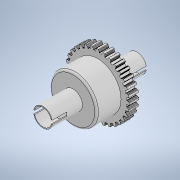
# Autodesk Inventor part: Дифференциал
Saved by Autodesk Inventor 2020 (Build 240168000, 168)
## iProperties
Created: 2021-05-23
Part Number: Дифференциал
Material: Типовые
Document SubType Name: Modeling
Designer: Антон
Density: 1 g/cm^3
Appearance: По умолчанию
Author: Антон
Autodesk Inventor part; units mm, degrees
ref_plane "YZ Plane" through (0, 0, 0) normal (1, 0, 0) x (0, 1, 0)
ref_plane "XZ Plane" through (0, 0, 0) normal (0, 1, 0) x (-1, 0, 0)
sketch "Эскиз1" plane through (0, 0, 0) normal (0, 0, 1) x (1, 0, 0)
  line L0 (32.4043, 17.9453) -> (32.4686, 17.9378)
  line L1 (32.4686, 17.9378) -> (32.5329, 17.9288)
  line L2 (32.5329, 17.9288) -> (32.6618, 17.9069)
  line L3 (32.6618, 17.9069) -> (32.9201, 17.8497)
  line L4 (32.9201, 17.8497) -> (33.1788, 17.7769)
  line L5 (33.1788, 17.7769) -> (33.4377, 17.69)
  line L6 (33.4377, 17.69) -> (33.6965, 17.5903)
  line L7 (33.6965, 17.5903) -> (33.9549, 17.4785)
  line L8 (33.9549, 17.4785) -> (33.9549, 16.4837)
  line L9 (33.9549, 16.4837) -> (33.6965, 16.3719)
  line L10 (33.6965, 16.3719) -> (33.4377, 16.2722)
  line L11 (33.4377, 16.2722) -> (33.1788, 16.1854)
  line L12 (33.1788, 16.1854) -> (32.9201, 16.1125)
  line L13 (32.9201, 16.1125) -> (32.6618, 16.0553)
  line L14 (32.6618, 16.0553) -> (32.5329, 16.0334)
  line L15 (32.5329, 16.0334) -> (32.4686, 16.0245)
  line L16 (32.4686, 16.0245) -> (32.4043, 16.017)
  line L17 (32.4043, 16.017) -> (32.2961, 14.9178)
  line L18 (32.2961, 14.9178) -> (32.3576, 14.8979)
  line L19 (32.3576, 14.8979) -> (32.419, 14.8766)
  line L20 (32.419, 14.8766) -> (32.5411, 14.83)
  line L21 (32.5411, 14.83) -> (32.7832, 14.7235)
  line L22 (32.7832, 14.7235) -> (33.0228, 14.6016)
  line L23 (33.0228, 14.6016) -> (33.2598, 14.4659)
  line L24 (33.2598, 14.4659) -> (33.4942, 14.3176)
  line L25 (33.4942, 14.3176) -> (33.7258, 14.1575)
  line L26 (33.7258, 14.1575) -> (33.5318, 13.1818)
  line L27 (33.5318, 13.1818) -> (33.2565, 13.1226)
  line L28 (33.2565, 13.1226) -> (32.9832, 13.0753)
  line L29 (32.9832, 13.0753) -> (32.7123, 13.0406)
  line L30 (32.7123, 13.0406) -> (32.4443, 13.0197)
  line L31 (32.4443, 13.0197) -> (32.1798, 13.0139)
  line L32 (32.1798, 13.0139) -> (32.0492, 13.0176)
  line L33 (32.0492, 13.0176) -> (31.9844, 13.0214)
  line L34 (31.9844, 13.0214) -> (31.9199, 13.0266)
  line L35 (31.9199, 13.0266) -> (31.5993, 11.9697)
  line L36 (31.5993, 11.9697) -> (31.6558, 11.9381)
  line L37 (31.6558, 11.9381) -> (31.7117, 11.9052)
  line L38 (31.7117, 11.9052) -> (31.8224, 11.8358)
  line L39 (31.8224, 11.8358) -> (32.0392, 11.684)
  line L40 (32.0392, 11.684) -> (32.2503, 11.5177)
  line L41 (32.2503, 11.5177) -> (32.4563, 11.3384)
  line L42 (32.4563, 11.3384) -> (32.6572, 11.1472)
  line L43 (32.6572, 11.1472) -> (32.8532, 10.9451)
  line L44 (32.8532, 10.9451) -> (32.4725, 10.026)
  line L45 (32.4725, 10.026) -> (32.191, 10.0216)
  line L46 (32.191, 10.0216) -> (31.9137, 10.0285)
  line L47 (31.9137, 10.0285) -> (31.6413, 10.0474)
  line L48 (31.6413, 10.0474) -> (31.3744, 10.0791)
  line L49 (31.3744, 10.0791) -> (31.1138, 10.125)
  line L50 (31.1138, 10.125) -> (30.9864, 10.1542)
  line L51 (30.9864, 10.1542) -> (30.9236, 10.1705)
  line L52 (30.9236, 10.1705) -> (30.8613, 10.1882)
  line L53 (30.8613, 10.1882) -> (30.3407, 9.2141)
  line L54 (30.3407, 9.2141) -> (30.3899, 9.1722)
  line L55 (30.3899, 9.1722) -> (30.4385, 9.129)
  line L56 (30.4385, 9.129) -> (30.5335, 9.0392)
  line L57 (30.5335, 9.0392) -> (30.7164, 8.8482)
  line L58 (30.7164, 8.8482) -> (30.8911, 8.6438)
  line L59 (30.8911, 8.6438) -> (31.0581, 8.4278)
  line L60 (31.0581, 8.4278) -> (31.2179, 8.2011)
  line L61 (31.2179, 8.2011) -> (31.3707, 7.9645)
  line L62 (31.3707, 7.9645) -> (30.818, 7.1374)
  line L63 (30.818, 7.1374) -> (30.541, 7.188)
  line L64 (30.541, 7.188) -> (30.2704, 7.2489)
  line L65 (30.2704, 7.2489) -> (30.0069, 7.3205)
  line L66 (30.0069, 7.3205) -> (29.7513, 7.4037)
  line L67 (29.7513, 7.4037) -> (29.5047, 7.4996)
  line L68 (29.5047, 7.4996) -> (29.3854, 7.553)
  line L69 (29.3854, 7.553) -> (29.327, 7.5813)
  line L70 (29.327, 7.5813) -> (29.2694, 7.6108)
  line L71 (29.2694, 7.6108) -> (28.5687, 6.757)
  line L72 (28.5687, 6.757) -> (28.6089, 6.7063)
  line L73 (28.6089, 6.7063) -> (28.648, 6.6545)
  line L74 (28.648, 6.6545) -> (28.7237, 6.5479)
  line L75 (28.7237, 6.5479) -> (28.8659, 6.3248)
  line L76 (28.8659, 6.3248) -> (28.9973, 6.0903)
  line L77 (28.9973, 6.0903) -> (29.119, 5.8458)
  line L78 (29.119, 5.8458) -> (29.2314, 5.5923)
  line L79 (29.2314, 5.5923) -> (29.3351, 5.3305)
  line L80 (29.3351, 5.3305) -> (28.6317, 4.6271)
  line L81 (28.6317, 4.6271) -> (28.3699, 4.7308)
  line L82 (28.3699, 4.7308) -> (28.1164, 4.8433)
  line L83 (28.1164, 4.8433) -> (27.8719, 4.9649)
  line L84 (27.8719, 4.9649) -> (27.6374, 5.0964)
  line L85 (27.6374, 5.0964) -> (27.4143, 5.2386)
  line L86 (27.4143, 5.2386) -> (27.3078, 5.3142)
  line L87 (27.3078, 5.3142) -> (27.256, 5.3534)
  line L88 (27.256, 5.3534) -> (27.2052, 5.3935)
  line L89 (27.2052, 5.3935) -> (26.3514, 4.6928)
  line L90 (26.3514, 4.6928) -> (26.3809, 4.6353)
  line L91 (26.3809, 4.6353) -> (26.4092, 4.5768)
  line L92 (26.4092, 4.5768) -> (26.4626, 4.4575)
  line L93 (26.4626, 4.4575) -> (26.5585, 4.211)
  line L94 (26.5585, 4.211) -> (26.6417, 3.9553)
  line L95 (26.6417, 3.9553) -> (26.7133, 3.6918)
  line L96 (26.7133, 3.6918) -> (26.7742, 3.4212)
  line L97 (26.7742, 3.4212) -> (26.8248, 3.1442)
  line L98 (26.8248, 3.1442) -> (25.9977, 2.5915)
  line L99 (25.9977, 2.5915) -> (25.7611, 2.7443)
  line L100 (25.7611, 2.7443) -> (25.5345, 2.9041)
  line L101 (25.5345, 2.9041) -> (25.3184, 3.0712)
  line L102 (25.3184, 3.0712) -> (25.1141, 3.2458)
  line L103 (25.1141, 3.2458) -> (24.923, 3.4288)
  line L104 (24.923, 3.4288) -> (24.8333, 3.5238)
  line L105 (24.8333, 3.5238) -> (24.7901, 3.5723)
  line L106 (24.7901, 3.5723) -> (24.7481, 3.6215)
  line L107 (24.7481, 3.6215) -> (23.7741, 3.1009)
  line L108 (23.7741, 3.1009) -> (23.7917, 3.0387)
  line L109 (23.7917, 3.0387) -> (23.8081, 2.9758)
  line L110 (23.8081, 2.9758) -> (23.8372, 2.8484)
  line L111 (23.8372, 2.8484) -> (23.8832, 2.5879)
  line L112 (23.8832, 2.5879) -> (23.9149, 2.3209)
  line L113 (23.9149, 2.3209) -> (23.9337, 2.0485)
  line L114 (23.9337, 2.0485) -> (23.9407, 1.7712)
  line L115 (23.9407, 1.7712) -> (23.9363, 1.4897)
  line L116 (23.9363, 1.4897) -> (23.0172, 1.109)
  line L117 (23.0172, 1.109) -> (22.815, 1.305)
  line L118 (22.815, 1.305) -> (22.6238, 1.5059)
  line L119 (22.6238, 1.5059) -> (22.4445, 1.7119)
  line L120 (22.4445, 1.7119) -> (22.2782, 1.9231)
  line L121 (22.2782, 1.9231) -> (22.1265, 2.1398)
  line L122 (22.1265, 2.1398) -> (22.057, 2.2505)
  line L123 (22.057, 2.2505) -> (22.0241, 2.3065)
  line L124 (22.0241, 2.3065) -> (21.9926, 2.363)
  line L125 (21.9926, 2.363) -> (20.9356, 2.0423)
  line L126 (20.9356, 2.0423) -> (20.9408, 1.9779)
  line L127 (20.9408, 1.9779) -> (20.9446, 1.913)
  line L128 (20.9446, 1.913) -> (20.9483, 1.7824)
  line L129 (20.9483, 1.7824) -> (20.9426, 1.5179)
  line L130 (20.9426, 1.5179) -> (20.9216, 1.2499)
  line L131 (20.9216, 1.2499) -> (20.8869, 0.979)
  line L132 (20.8869, 0.979) -> (20.8396, 0.7058)
  line L133 (20.8396, 0.7058) -> (20.7804, 0.4305)
  line L134 (20.7804, 0.4305) -> (19.8047, 0.2364)
  line L135 (19.8047, 0.2364) -> (19.6446, 0.4681)
  line L136 (19.6446, 0.4681) -> (19.4963, 0.7024)
  line L137 (19.4963, 0.7024) -> (19.3607, 0.9394)
  line L138 (19.3607, 0.9394) -> (19.2387, 1.179)
  line L139 (19.2387, 1.179) -> (19.1322, 1.4211)
  line L140 (19.1322, 1.4211) -> (19.0857, 1.5433)
  line L141 (19.0857, 1.5433) -> (19.0643, 1.6046)
  line L142 (19.0643, 1.6046) -> (19.0444, 1.6662)
  line L143 (19.0444, 1.6662) -> (17.9453, 1.5579)
  line L144 (17.9453, 1.5579) -> (17.9378, 1.4937)
  line L145 (17.9378, 1.4937) -> (17.9288, 1.4293)
  line L146 (17.9288, 1.4293) -> (17.9069, 1.3005)
  line L147 (17.9069, 1.3005) -> (17.8497, 1.0422)
  line L148 (17.8497, 1.0422) -> (17.7769, 0.7834)
  line L149 (17.7769, 0.7834) -> (17.69, 0.5245)
  line L150 (17.69, 0.5245) -> (17.5903, 0.2657)
  line L151 (17.5903, 0.2657) -> (17.4785, 0.0073)
  line L152 (17.4785, 0.0073) -> (16.4837, 0.0073)
  line L153 (16.4837, 0.0073) -> (16.3719, 0.2657)
  line L154 (16.3719, 0.2657) -> (16.2722, 0.5245)
  line L155 (16.2722, 0.5245) -> (16.1854, 0.7834)
  line L156 (16.1854, 0.7834) -> (16.1125, 1.0422)
  line L157 (16.1125, 1.0422) -> (16.0553, 1.3005)
  line L158 (16.0553, 1.3005) -> (16.0334, 1.4293)
  line L159 (16.0334, 1.4293) -> (16.0245, 1.4937)
  line L160 (16.0245, 1.4937) -> (16.017, 1.5579)
  line L161 (16.017, 1.5579) -> (14.9178, 1.6662)
  line L162 (14.9178, 1.6662) -> (14.8979, 1.6046)
  line L163 (14.8979, 1.6046) -> (14.8766, 1.5433)
  line L164 (14.8766, 1.5433) -> (14.83, 1.4211)
  line L165 (14.83, 1.4211) -> (14.7235, 1.179)
  line L166 (14.7235, 1.179) -> (14.6016, 0.9394)
  line L167 (14.6016, 0.9394) -> (14.4659, 0.7024)
  line L168 (14.4659, 0.7024) -> (14.3176, 0.4681)
  line L169 (14.3176, 0.4681) -> (14.1575, 0.2364)
  line L170 (14.1575, 0.2364) -> (13.1818, 0.4305)
  line L171 (13.1818, 0.4305) -> (13.1226, 0.7058)
  line L172 (13.1226, 0.7058) -> (13.0753, 0.979)
  line L173 (13.0753, 0.979) -> (13.0406, 1.2499)
  line L174 (13.0406, 1.2499) -> (13.0197, 1.5179)
  line L175 (13.0197, 1.5179) -> (13.0139, 1.7824)
  line L176 (13.0139, 1.7824) -> (13.0176, 1.913)
  line L177 (13.0176, 1.913) -> (13.0214, 1.9779)
  line L178 (13.0214, 1.9779) -> (13.0266, 2.0423)
  line L179 (13.0266, 2.0423) -> (11.9697, 2.363)
  line L180 (11.9697, 2.363) -> (11.9381, 2.3065)
  line L181 (11.9381, 2.3065) -> (11.9052, 2.2505)
  line L182 (11.9052, 2.2505) -> (11.8358, 2.1398)
  line L183 (11.8358, 2.1398) -> (11.684, 1.9231)
  line L184 (11.684, 1.9231) -> (11.5177, 1.7119)
  line L185 (11.5177, 1.7119) -> (11.3384, 1.5059)
  line L186 (11.3384, 1.5059) -> (11.1472, 1.305)
  line L187 (11.1472, 1.305) -> (10.9451, 1.109)
  line L188 (10.9451, 1.109) -> (10.026, 1.4897)
  line L189 (10.026, 1.4897) -> (10.0216, 1.7712)
  line L190 (10.0216, 1.7712) -> (10.0285, 2.0485)
  line L191 (10.0285, 2.0485) -> (10.0474, 2.3209)
  line L192 (10.0474, 2.3209) -> (10.0791, 2.5879)
  line L193 (10.0791, 2.5879) -> (10.125, 2.8484)
  line L194 (10.125, 2.8484) -> (10.1542, 2.9758)
  line L195 (10.1542, 2.9758) -> (10.1705, 3.0387)
  line L196 (10.1705, 3.0387) -> (10.1882, 3.1009)
  line L197 (10.1882, 3.1009) -> (9.2141, 3.6215)
  line L198 (9.2141, 3.6215) -> (9.1722, 3.5723)
  line L199 (9.1722, 3.5723) -> (9.129, 3.5238)
  line L200 (9.129, 3.5238) -> (9.0392, 3.4288)
  line L201 (9.0392, 3.4288) -> (8.8482, 3.2458)
  line L202 (8.8482, 3.2458) -> (8.6438, 3.0712)
  line L203 (8.6438, 3.0712) -> (8.4278, 2.9041)
  line L204 (8.4278, 2.9041) -> (8.2011, 2.7443)
  line L205 (8.2011, 2.7443) -> (7.9645, 2.5915)
  line L206 (7.9645, 2.5915) -> (7.1374, 3.1442)
  line L207 (7.1374, 3.1442) -> (7.188, 3.4212)
  line L208 (7.188, 3.4212) -> (7.2489, 3.6918)
  line L209 (7.2489, 3.6918) -> (7.3205, 3.9553)
  line L210 (7.3205, 3.9553) -> (7.4037, 4.211)
  line L211 (7.4037, 4.211) -> (7.4996, 4.4575)
  line L212 (7.4996, 4.4575) -> (7.553, 4.5768)
  line L213 (7.553, 4.5768) -> (7.5813, 4.6353)
  line L214 (7.5813, 4.6353) -> (7.6108, 4.6928)
  line L215 (7.6108, 4.6928) -> (6.757, 5.3935)
  line L216 (6.757, 5.3935) -> (6.7063, 5.3534)
  line L217 (6.7063, 5.3534) -> (6.6545, 5.3142)
  line L218 (6.6545, 5.3142) -> (6.5479, 5.2386)
  line L219 (6.5479, 5.2386) -> (6.3248, 5.0964)
  line L220 (6.3248, 5.0964) -> (6.0903, 4.9649)
  line L221 (6.0903, 4.9649) -> (5.8458, 4.8433)
  line L222 (5.8458, 4.8433) -> (5.5923, 4.7308)
  line L223 (5.5923, 4.7308) -> (5.3305, 4.6271)
  line L224 (5.3305, 4.6271) -> (4.6271, 5.3305)
  line L225 (4.6271, 5.3305) -> (4.7308, 5.5923)
  line L226 (4.7308, 5.5923) -> (4.8433, 5.8458)
  line L227 (4.8433, 5.8458) -> (4.9649, 6.0903)
  line L228 (4.9649, 6.0903) -> (5.0964, 6.3248)
  line L229 (5.0964, 6.3248) -> (5.2386, 6.5479)
  line L230 (5.2386, 6.5479) -> (5.3142, 6.6545)
  line L231 (5.3142, 6.6545) -> (5.3534, 6.7063)
  line L232 (5.3534, 6.7063) -> (5.3935, 6.757)
  line L233 (5.3935, 6.757) -> (4.6928, 7.6108)
  line L234 (4.6928, 7.6108) -> (4.6353, 7.5813)
  line L235 (4.6353, 7.5813) -> (4.5768, 7.553)
  line L236 (4.5768, 7.553) -> (4.4575, 7.4996)
  line L237 (4.4575, 7.4996) -> (4.211, 7.4037)
  line L238 (4.211, 7.4037) -> (3.9553, 7.3205)
  line L239 (3.9553, 7.3205) -> (3.6918, 7.2489)
  line L240 (3.6918, 7.2489) -> (3.4212, 7.188)
  line L241 (3.4212, 7.188) -> (3.1442, 7.1374)
  line L242 (3.1442, 7.1374) -> (2.5915, 7.9645)
  line L243 (2.5915, 7.9645) -> (2.7443, 8.2011)
  line L244 (2.7443, 8.2011) -> (2.9041, 8.4278)
  line L245 (2.9041, 8.4278) -> (3.0712, 8.6438)
  line L246 (3.0712, 8.6438) -> (3.2458, 8.8482)
  line L247 (3.2458, 8.8482) -> (3.4288, 9.0392)
  line L248 (3.4288, 9.0392) -> (3.5238, 9.129)
  line L249 (3.5238, 9.129) -> (3.5723, 9.1722)
  line L250 (3.5723, 9.1722) -> (3.6215, 9.2141)
  line L251 (3.6215, 9.2141) -> (3.1009, 10.1882)
  line L252 (3.1009, 10.1882) -> (3.0387, 10.1705)
  line L253 (3.0387, 10.1705) -> (2.9758, 10.1542)
  line L254 (2.9758, 10.1542) -> (2.8484, 10.125)
  line L255 (2.8484, 10.125) -> (2.5879, 10.0791)
  line L256 (2.5879, 10.0791) -> (2.3209, 10.0474)
  line L257 (2.3209, 10.0474) -> (2.0485, 10.0285)
  line L258 (2.0485, 10.0285) -> (1.7712, 10.0216)
  line L259 (1.7712, 10.0216) -> (1.4897, 10.026)
  line L260 (1.4897, 10.026) -> (1.109, 10.9451)
  line L261 (1.109, 10.9451) -> (1.305, 11.1472)
  line L262 (1.305, 11.1472) -> (1.5059, 11.3384)
  line L263 (1.5059, 11.3384) -> (1.7119, 11.5177)
  line L264 (1.7119, 11.5177) -> (1.9231, 11.684)
  line L265 (1.9231, 11.684) -> (2.1398, 11.8358)
  line L266 (2.1398, 11.8358) -> (2.2505, 11.9052)
  line L267 (2.2505, 11.9052) -> (2.3065, 11.9381)
  line L268 (2.3065, 11.9381) -> (2.363, 11.9697)
  line L269 (2.363, 11.9697) -> (2.0423, 13.0266)
  line L270 (2.0423, 13.0266) -> (1.9779, 13.0214)
  line L271 (1.9779, 13.0214) -> (1.913, 13.0176)
  line L272 (1.913, 13.0176) -> (1.7824, 13.0139)
  line L273 (1.7824, 13.0139) -> (1.5179, 13.0197)
  line L274 (1.5179, 13.0197) -> (1.2499, 13.0406)
  line L275 (1.2499, 13.0406) -> (0.979, 13.0753)
  line L276 (0.979, 13.0753) -> (0.7058, 13.1226)
  line L277 (0.7058, 13.1226) -> (0.4305, 13.1818)
  line L278 (0.4305, 13.1818) -> (0.2364, 14.1575)
  line L279 (0.2364, 14.1575) -> (0.4681, 14.3176)
  line L280 (0.4681, 14.3176) -> (0.7024, 14.4659)
  line L281 (0.7024, 14.4659) -> (0.9394, 14.6016)
  line L282 (0.9394, 14.6016) -> (1.179, 14.7235)
  line L283 (1.179, 14.7235) -> (1.4211, 14.83)
  line L284 (1.4211, 14.83) -> (1.5433, 14.8766)
  line L285 (1.5433, 14.8766) -> (1.6046, 14.8979)
  line L286 (1.6046, 14.8979) -> (1.6662, 14.9178)
  line L287 (1.6662, 14.9178) -> (1.5579, 16.017)
  line L288 (1.5579, 16.017) -> (1.4937, 16.0245)
  line L289 (1.4937, 16.0245) -> (1.4293, 16.0334)
  line L290 (1.4293, 16.0334) -> (1.3005, 16.0553)
  line L291 (1.3005, 16.0553) -> (1.0422, 16.1125)
  line L292 (1.0422, 16.1125) -> (0.7834, 16.1854)
  line L293 (0.7834, 16.1854) -> (0.5245, 16.2722)
  line L294 (0.5245, 16.2722) -> (0.2657, 16.3719)
  line L295 (0.2657, 16.3719) -> (0.0073, 16.4837)
  line L296 (0.0073, 16.4837) -> (0.0073, 17.4785)
  line L297 (0.0073, 17.4785) -> (0.2657, 17.5903)
  line L298 (0.2657, 17.5903) -> (0.5245, 17.69)
  line L299 (0.5245, 17.69) -> (0.7834, 17.7769)
  line L300 (0.7834, 17.7769) -> (1.0422, 17.8497)
  line L301 (1.0422, 17.8497) -> (1.3005, 17.9069)
  line L302 (1.3005, 17.9069) -> (1.4293, 17.9288)
  line L303 (1.4293, 17.9288) -> (1.4937, 17.9378)
  line L304 (1.4937, 17.9378) -> (1.5579, 17.9453)
  line L305 (1.5579, 17.9453) -> (1.6662, 19.0444)
  line L306 (1.6662, 19.0444) -> (1.6046, 19.0643)
  line L307 (1.6046, 19.0643) -> (1.5433, 19.0857)
  line L308 (1.5433, 19.0857) -> (1.4211, 19.1322)
  line L309 (1.4211, 19.1322) -> (1.179, 19.2387)
  line L310 (1.179, 19.2387) -> (0.9394, 19.3607)
  line L311 (0.9394, 19.3607) -> (0.7024, 19.4963)
  line L312 (0.7024, 19.4963) -> (0.4681, 19.6446)
  line L313 (0.4681, 19.6446) -> (0.2364, 19.8047)
  line L314 (0.2364, 19.8047) -> (0.4305, 20.7804)
  line L315 (0.4305, 20.7804) -> (0.7058, 20.8396)
  line L316 (0.7058, 20.8396) -> (0.979, 20.8869)
  line L317 (0.979, 20.8869) -> (1.2499, 20.9216)
  line L318 (1.2499, 20.9216) -> (1.5179, 20.9426)
  line L319 (1.5179, 20.9426) -> (1.7824, 20.9483)
  line L320 (1.7824, 20.9483) -> (1.913, 20.9446)
  line L321 (1.913, 20.9446) -> (1.9779, 20.9408)
  line L322 (1.9779, 20.9408) -> (2.0423, 20.9356)
  line L323 (2.0423, 20.9356) -> (2.363, 21.9926)
  line L324 (2.363, 21.9926) -> (2.3065, 22.0241)
  line L325 (2.3065, 22.0241) -> (2.2505, 22.057)
  line L326 (2.2505, 22.057) -> (2.1398, 22.1265)
  line L327 (2.1398, 22.1265) -> (1.9231, 22.2782)
  line L328 (1.9231, 22.2782) -> (1.7119, 22.4445)
  line L329 (1.7119, 22.4445) -> (1.5059, 22.6238)
  line L330 (1.5059, 22.6238) -> (1.305, 22.815)
  line L331 (1.305, 22.815) -> (1.109, 23.0172)
  line L332 (1.109, 23.0172) -> (1.4897, 23.9363)
  line L333 (1.4897, 23.9363) -> (1.7712, 23.9407)
  line L334 (1.7712, 23.9407) -> (2.0485, 23.9337)
  line L335 (2.0485, 23.9337) -> (2.3209, 23.9149)
  line L336 (2.3209, 23.9149) -> (2.5879, 23.8832)
  line L337 (2.5879, 23.8832) -> (2.8484, 23.8372)
  line L338 (2.8484, 23.8372) -> (2.9758, 23.8081)
  line L339 (2.9758, 23.8081) -> (3.0387, 23.7917)
  line L340 (3.0387, 23.7917) -> (3.1009, 23.7741)
  line L341 (3.1009, 23.7741) -> (3.6215, 24.7481)
  line L342 (3.6215, 24.7481) -> (3.5723, 24.7901)
  line L343 (3.5723, 24.7901) -> (3.5238, 24.8333)
  line L344 (3.5238, 24.8333) -> (3.4288, 24.923)
  line L345 (3.4288, 24.923) -> (3.2458, 25.1141)
  line L346 (3.2458, 25.1141) -> (3.0712, 25.3184)
  line L347 (3.0712, 25.3184) -> (2.9041, 25.5345)
  line L348 (2.9041, 25.5345) -> (2.7443, 25.7611)
  line L349 (2.7443, 25.7611) -> (2.5915, 25.9977)
  line L350 (2.5915, 25.9977) -> (3.1442, 26.8248)
  line L351 (3.1442, 26.8248) -> (3.4212, 26.7742)
  line L352 (3.4212, 26.7742) -> (3.6918, 26.7133)
  line L353 (3.6918, 26.7133) -> (3.9553, 26.6417)
  line L354 (3.9553, 26.6417) -> (4.211, 26.5585)
  line L355 (4.211, 26.5585) -> (4.4575, 26.4626)
  line L356 (4.4575, 26.4626) -> (4.5768, 26.4092)
  line L357 (4.5768, 26.4092) -> (4.6353, 26.3809)
  line L358 (4.6353, 26.3809) -> (4.6928, 26.3514)
  line L359 (4.6928, 26.3514) -> (5.3935, 27.2052)
  line L360 (5.3935, 27.2052) -> (5.3534, 27.256)
  line L361 (5.3534, 27.256) -> (5.3142, 27.3078)
  line L362 (5.3142, 27.3078) -> (5.2386, 27.4143)
  line L363 (5.2386, 27.4143) -> (5.0964, 27.6374)
  line L364 (5.0964, 27.6374) -> (4.9649, 27.8719)
  line L365 (4.9649, 27.8719) -> (4.8433, 28.1164)
  line L366 (4.8433, 28.1164) -> (4.7308, 28.3699)
  line L367 (4.7308, 28.3699) -> (4.6271, 28.6317)
  line L368 (4.6271, 28.6317) -> (5.3305, 29.3351)
  line L369 (5.3305, 29.3351) -> (5.5923, 29.2314)
  line L370 (5.5923, 29.2314) -> (5.8458, 29.119)
  line L371 (5.8458, 29.119) -> (6.0903, 28.9973)
  line L372 (6.0903, 28.9973) -> (6.3248, 28.8659)
  line L373 (6.3248, 28.8659) -> (6.5479, 28.7237)
  line L374 (6.5479, 28.7237) -> (6.6545, 28.648)
  line L375 (6.6545, 28.648) -> (6.7063, 28.6089)
  line L376 (6.7063, 28.6089) -> (6.757, 28.5687)
  line L377 (6.757, 28.5687) -> (7.6108, 29.2694)
  line L378 (7.6108, 29.2694) -> (7.5813, 29.327)
  line L379 (7.5813, 29.327) -> (7.553, 29.3854)
  line L380 (7.553, 29.3854) -> (7.4996, 29.5047)
  line L381 (7.4996, 29.5047) -> (7.4037, 29.7513)
  line L382 (7.4037, 29.7513) -> (7.3205, 30.0069)
  line L383 (7.3205, 30.0069) -> (7.2489, 30.2704)
  line L384 (7.2489, 30.2704) -> (7.188, 30.541)
  line L385 (7.188, 30.541) -> (7.1374, 30.818)
  line L386 (7.1374, 30.818) -> (7.9645, 31.3707)
  line L387 (7.9645, 31.3707) -> (8.2011, 31.2179)
  line L388 (8.2011, 31.2179) -> (8.4278, 31.0581)
  line L389 (8.4278, 31.0581) -> (8.6438, 30.8911)
  line L390 (8.6438, 30.8911) -> (8.8482, 30.7164)
  line L391 (8.8482, 30.7164) -> (9.0392, 30.5335)
  line L392 (9.0392, 30.5335) -> (9.129, 30.4385)
  line L393 (9.129, 30.4385) -> (9.1722, 30.3899)
  line L394 (9.1722, 30.3899) -> (9.2141, 30.3407)
  line L395 (9.2141, 30.3407) -> (10.1882, 30.8613)
  line L396 (10.1882, 30.8613) -> (10.1705, 30.9236)
  line L397 (10.1705, 30.9236) -> (10.1542, 30.9864)
  line L398 (10.1542, 30.9864) -> (10.125, 31.1138)
  line L399 (10.125, 31.1138) -> (10.0791, 31.3744)
  line L400 (10.0791, 31.3744) -> (10.0474, 31.6413)
  line L401 (10.0474, 31.6413) -> (10.0285, 31.9137)
  line L402 (10.0285, 31.9137) -> (10.0216, 32.191)
  line L403 (10.0216, 32.191) -> (10.026, 32.4725)
  line L404 (10.026, 32.4725) -> (10.9451, 32.8532)
  line L405 (10.9451, 32.8532) -> (11.1472, 32.6572)
  line L406 (11.1472, 32.6572) -> (11.3384, 32.4563)
  line L407 (11.3384, 32.4563) -> (11.5177, 32.2503)
  line L408 (11.5177, 32.2503) -> (11.684, 32.0392)
  line L409 (11.684, 32.0392) -> (11.8358, 31.8224)
  line L410 (11.8358, 31.8224) -> (11.9052, 31.7117)
  line L411 (11.9052, 31.7117) -> (11.9381, 31.6558)
  line L412 (11.9381, 31.6558) -> (11.9697, 31.5993)
  line L413 (11.9697, 31.5993) -> (13.0266, 31.9199)
  line L414 (13.0266, 31.9199) -> (13.0214, 31.9844)
  line L415 (13.0214, 31.9844) -> (13.0176, 32.0492)
  line L416 (13.0176, 32.0492) -> (13.0139, 32.1798)
  line L417 (13.0139, 32.1798) -> (13.0197, 32.4443)
  line L418 (13.0197, 32.4443) -> (13.0406, 32.7123)
  line L419 (13.0406, 32.7123) -> (13.0753, 32.9832)
  line L420 (13.0753, 32.9832) -> (13.1226, 33.2565)
  line L421 (13.1226, 33.2565) -> (13.1818, 33.5318)
  line L422 (13.1818, 33.5318) -> (14.1575, 33.7258)
  line L423 (14.1575, 33.7258) -> (14.3176, 33.4942)
  line L424 (14.3176, 33.4942) -> (14.4659, 33.2598)
  line L425 (14.4659, 33.2598) -> (14.6016, 33.0228)
  line L426 (14.6016, 33.0228) -> (14.7235, 32.7832)
  line L427 (14.7235, 32.7832) -> (14.83, 32.5411)
  line L428 (14.83, 32.5411) -> (14.8766, 32.419)
  line L429 (14.8766, 32.419) -> (14.8979, 32.3576)
  line L430 (14.8979, 32.3576) -> (14.9178, 32.2961)
  line L431 (14.9178, 32.2961) -> (16.017, 32.4043)
  line L432 (16.017, 32.4043) -> (16.0245, 32.4686)
  line L433 (16.0245, 32.4686) -> (16.0334, 32.5329)
  line L434 (16.0334, 32.5329) -> (16.0553, 32.6618)
  line L435 (16.0553, 32.6618) -> (16.1125, 32.9201)
  line L436 (16.1125, 32.9201) -> (16.1854, 33.1788)
  line L437 (16.1854, 33.1788) -> (16.2722, 33.4377)
  line L438 (16.2722, 33.4377) -> (16.3719, 33.6965)
  line L439 (16.3719, 33.6965) -> (16.4837, 33.9549)
  line L440 (16.4837, 33.9549) -> (17.4785, 33.9549)
  line L441 (17.4785, 33.9549) -> (17.5903, 33.6965)
  line L442 (17.5903, 33.6965) -> (17.69, 33.4377)
  line L443 (17.69, 33.4377) -> (17.7769, 33.1788)
  line L444 (17.7769, 33.1788) -> (17.8497, 32.9201)
  line L445 (17.8497, 32.9201) -> (17.9069, 32.6618)
  line L446 (17.9069, 32.6618) -> (17.9288, 32.5329)
  line L447 (17.9288, 32.5329) -> (17.9378, 32.4686)
  line L448 (17.9378, 32.4686) -> (17.9453, 32.4043)
  line L449 (17.9453, 32.4043) -> (19.0444, 32.2961)
  line L450 (19.0444, 32.2961) -> (19.0643, 32.3576)
  line L451 (19.0643, 32.3576) -> (19.0857, 32.419)
  line L452 (19.0857, 32.419) -> (19.1322, 32.5411)
  line L453 (19.1322, 32.5411) -> (19.2387, 32.7832)
  line L454 (19.2387, 32.7832) -> (19.3607, 33.0228)
  line L455 (19.3607, 33.0228) -> (19.4963, 33.2598)
  line L456 (19.4963, 33.2598) -> (19.6446, 33.4942)
  line L457 (19.6446, 33.4942) -> (19.8047, 33.7258)
  line L458 (19.8047, 33.7258) -> (20.7804, 33.5318)
  line L459 (20.7804, 33.5318) -> (20.8396, 33.2565)
  line L460 (20.8396, 33.2565) -> (20.8869, 32.9832)
  line L461 (20.8869, 32.9832) -> (20.9216, 32.7123)
  line L462 (20.9216, 32.7123) -> (20.9426, 32.4443)
  line L463 (20.9426, 32.4443) -> (20.9483, 32.1798)
  line L464 (20.9483, 32.1798) -> (20.9446, 32.0492)
  line L465 (20.9446, 32.0492) -> (20.9408, 31.9844)
  line L466 (20.9408, 31.9844) -> (20.9356, 31.9199)
  line L467 (20.9356, 31.9199) -> (21.9926, 31.5993)
  line L468 (21.9926, 31.5993) -> (22.0241, 31.6558)
  line L469 (22.0241, 31.6558) -> (22.057, 31.7117)
  line L470 (22.057, 31.7117) -> (22.1265, 31.8224)
  line L471 (22.1265, 31.8224) -> (22.2782, 32.0392)
  line L472 (22.2782, 32.0392) -> (22.4445, 32.2503)
  line L473 (22.4445, 32.2503) -> (22.6238, 32.4563)
  line L474 (22.6238, 32.4563) -> (22.815, 32.6572)
  line L475 (22.815, 32.6572) -> (23.0172, 32.8532)
  line L476 (23.0172, 32.8532) -> (23.9363, 32.4725)
  line L477 (23.9363, 32.4725) -> (23.9407, 32.191)
  line L478 (23.9407, 32.191) -> (23.9337, 31.9137)
  line L479 (23.9337, 31.9137) -> (23.9149, 31.6413)
  line L480 (23.9149, 31.6413) -> (23.8832, 31.3744)
  line L481 (23.8832, 31.3744) -> (23.8372, 31.1138)
  line L482 (23.8372, 31.1138) -> (23.8081, 30.9864)
  line L483 (23.8081, 30.9864) -> (23.7917, 30.9236)
  line L484 (23.7917, 30.9236) -> (23.7741, 30.8613)
  line L485 (23.7741, 30.8613) -> (24.7481, 30.3407)
  line L486 (24.7481, 30.3407) -> (24.7901, 30.3899)
  line L487 (24.7901, 30.3899) -> (24.8333, 30.4385)
  line L488 (24.8333, 30.4385) -> (24.923, 30.5335)
  line L489 (24.923, 30.5335) -> (25.1141, 30.7164)
  line L490 (25.1141, 30.7164) -> (25.3184, 30.8911)
  line L491 (25.3184, 30.8911) -> (25.5345, 31.0581)
  line L492 (25.5345, 31.0581) -> (25.7611, 31.2179)
  line L493 (25.7611, 31.2179) -> (25.9977, 31.3707)
  line L494 (25.9977, 31.3707) -> (26.8248, 30.818)
  line L495 (26.8248, 30.818) -> (26.7742, 30.541)
  line L496 (26.7742, 30.541) -> (26.7133, 30.2704)
  line L497 (26.7133, 30.2704) -> (26.6417, 30.0069)
  line L498 (26.6417, 30.0069) -> (26.5585, 29.7513)
  line L499 (26.5585, 29.7513) -> (26.4626, 29.5047)
  line L500 (26.4626, 29.5047) -> (26.4092, 29.3854)
  line L501 (26.4092, 29.3854) -> (26.3809, 29.327)
  line L502 (26.3809, 29.327) -> (26.3514, 29.2694)
  line L503 (26.3514, 29.2694) -> (27.2052, 28.5687)
  line L504 (27.2052, 28.5687) -> (27.256, 28.6089)
  line L505 (27.256, 28.6089) -> (27.3078, 28.648)
  line L506 (27.3078, 28.648) -> (27.4143, 28.7237)
  line L507 (27.4143, 28.7237) -> (27.6374, 28.8659)
  line L508 (27.6374, 28.8659) -> (27.8719, 28.9973)
  line L509 (27.8719, 28.9973) -> (28.1164, 29.119)
  line L510 (28.1164, 29.119) -> (28.3699, 29.2314)
  line L511 (28.3699, 29.2314) -> (28.6317, 29.3351)
  line L512 (28.6317, 29.3351) -> (29.3351, 28.6317)
  line L513 (29.3351, 28.6317) -> (29.2314, 28.3699)
  line L514 (29.2314, 28.3699) -> (29.119, 28.1164)
  line L515 (29.119, 28.1164) -> (28.9973, 27.8719)
  line L516 (28.9973, 27.8719) -> (28.8659, 27.6374)
  line L517 (28.8659, 27.6374) -> (28.7237, 27.4143)
  line L518 (28.7237, 27.4143) -> (28.648, 27.3078)
  line L519 (28.648, 27.3078) -> (28.6089, 27.256)
  line L520 (28.6089, 27.256) -> (28.5687, 27.2052)
  line L521 (28.5687, 27.2052) -> (29.2694, 26.3514)
  line L522 (29.2694, 26.3514) -> (29.327, 26.3809)
  line L523 (29.327, 26.3809) -> (29.3854, 26.4092)
  line L524 (29.3854, 26.4092) -> (29.5047, 26.4626)
  line L525 (29.5047, 26.4626) -> (29.7513, 26.5585)
  line L526 (29.7513, 26.5585) -> (30.0069, 26.6417)
  line L527 (30.0069, 26.6417) -> (30.2704, 26.7133)
  line L528 (30.2704, 26.7133) -> (30.541, 26.7742)
  line L529 (30.541, 26.7742) -> (30.818, 26.8248)
  line L530 (30.818, 26.8248) -> (31.3707, 25.9977)
  line L531 (31.3707, 25.9977) -> (31.2179, 25.7611)
  line L532 (31.2179, 25.7611) -> (31.0581, 25.5345)
  line L533 (31.0581, 25.5345) -> (30.8911, 25.3184)
  line L534 (30.8911, 25.3184) -> (30.7164, 25.1141)
  line L535 (30.7164, 25.1141) -> (30.5335, 24.923)
  line L536 (30.5335, 24.923) -> (30.4385, 24.8333)
  line L537 (30.4385, 24.8333) -> (30.3899, 24.7901)
  line L538 (30.3899, 24.7901) -> (30.3407, 24.7481)
  line L539 (30.3407, 24.7481) -> (30.8613, 23.7741)
  line L540 (30.8613, 23.7741) -> (30.9236, 23.7917)
  line L541 (30.9236, 23.7917) -> (30.9864, 23.8081)
  line L542 (30.9864, 23.8081) -> (31.1138, 23.8372)
  line L543 (31.1138, 23.8372) -> (31.3744, 23.8832)
  line L544 (31.3744, 23.8832) -> (31.6413, 23.9149)
  line L545 (31.6413, 23.9149) -> (31.9137, 23.9337)
  line L546 (31.9137, 23.9337) -> (32.191, 23.9407)
  line L547 (32.191, 23.9407) -> (32.4725, 23.9363)
  line L548 (32.4725, 23.9363) -> (32.8532, 23.0172)
  line L549 (32.8532, 23.0172) -> (32.6572, 22.815)
  line L550 (32.6572, 22.815) -> (32.4563, 22.6238)
  line L551 (32.4563, 22.6238) -> (32.2503, 22.4445)
  line L552 (32.2503, 22.4445) -> (32.0392, 22.2782)
  line L553 (32.0392, 22.2782) -> (31.8224, 22.1265)
  line L554 (31.8224, 22.1265) -> (31.7117, 22.057)
  line L555 (31.7117, 22.057) -> (31.6558, 22.0241)
  line L556 (31.6558, 22.0241) -> (31.5993, 21.9926)
  line L557 (31.5993, 21.9926) -> (31.9199, 20.9356)
  line L558 (31.9199, 20.9356) -> (31.9844, 20.9408)
  line L559 (31.9844, 20.9408) -> (32.0492, 20.9446)
  line L560 (32.0492, 20.9446) -> (32.1798, 20.9483)
  line L561 (32.1798, 20.9483) -> (32.4443, 20.9426)
  line L562 (32.4443, 20.9426) -> (32.7123, 20.9216)
  line L563 (32.7123, 20.9216) -> (32.9832, 20.8869)
  line L564 (32.9832, 20.8869) -> (33.2565, 20.8396)
  line L565 (33.2565, 20.8396) -> (33.5318, 20.7804)
  line L566 (33.5318, 20.7804) -> (33.7258, 19.8047)
  line L567 (33.7258, 19.8047) -> (33.4942, 19.6446)
  line L568 (33.4942, 19.6446) -> (33.2598, 19.4963)
  line L569 (33.2598, 19.4963) -> (33.0228, 19.3607)
  line L570 (33.0228, 19.3607) -> (32.7832, 19.2387)
  line L571 (32.7832, 19.2387) -> (32.5411, 19.1322)
  line L572 (32.5411, 19.1322) -> (32.419, 19.0857)
  line L573 (32.419, 19.0857) -> (32.3576, 19.0643)
  line L574 (32.3576, 19.0643) -> (32.2961, 19.0444)
  line L575 (32.2961, 19.0444) -> (32.4043, 17.9453)
  circle A0 centre (16.9811, 16.9811) radius 0.5
  line L576 (11.3207, 16.9811) -> (22.6415, 16.9811)
  line L577 (16.9811, 11.3207) -> (16.9811, 22.6415)
  point P0 (0, 0)
  point P1 (17.4785, 0.0073)
  point P2 (0.0073, 16.4837)
  constraints: 1156 end point, 1 centre point
extrude "Выдавливание1" add sketch "Эскиз1" along normal blind 5 contours L0 L1 L2 L3 L4 L5 L6 L7 L8 L9 L10 L11 L12 L13 L14 L15 L16 L17 L18 L19 L20 L21 L22 L23 L24 L25 L26 L27 L28 L29 L30 L31 L32 L33 L34 L35 L36 L37 L38 L39 L40 L41 L42 L43 L44 L45 L46 L47 L48 L49 L50 L51 L52 L53 L54 L55 L56 L57 L58 L59 L60 L61 L62 L63 L64 L65 L66 L67 L68 L69 L70 L71 L72 L73 L74 L75 L76 L77 L78 L79 L80 L81 L82 L83 L84 L85 L86 L87 L88 L89 L90 L91 L92 L93 L94 L95 L96 L97 L98 L99 L100 L101 L102 L103 L104 L105 L106 L107 L108 L109 L110 L111 L112 L113 L114 L115 L116 L117 L118 L119 L120 L121 L122 L123 L124 L125 L126 L127 L128 L129 L130 L131 L132 L133 L134 L135 L136 L137 L138 L139 L140 L141 L142 L143 L144 L145 L146 L147 L148 L149 L150 L151 L152 L153 L154 L155 L156 L157 L158 L159 L160 L161 L162 L163 L164 L165 L166 L167 L168 L169 L170 L171 L172 L173 L174 L175 L176 L177 L178 L179 L180 L181 L182 L183 L184 L185 L186 L187 L188 L189 L190 L191 L192 L193 L194 L195 L196 L197 L198 L199 L200 L201 L202 L203 L204 L205 L206 L207 L208 L209 L210 L211 L212 L213 L214 L215 L216 L217 L218 L219 L220 L221 L222 L223 L224 L225 L226 L227 L228 L229 L230 L231 L232 L233 L234 L235 L236 L237 L238 L239 L240 L241 L242 L243 L244 L245 L246 L247 L248 L249 L250 L251 L252 L253 L254 L255 L256 L257 L258 L259 L260 L261 L262 L263 L264 L265 L266 L267 L268 L269 L270 L271 L272 L273 L274 L275 L276 L277 L278 L279 L280 L281 L282 L283 L284 L285 L286 L287 L288 L289 L290 L291 L292 L293 L294 L295 L296 L297 L298 L299 L300 L301 L302 L303 L304 L305 L306 L307 L308 L309 L310 L311 L312 L313 L314 L315 L316 L317 L318 L319 L320 L321 L322 L323 L324 L325 L326 L327 L328 L329 L330 L331 L332 L333 L334 L335 L336 L337 L338 L339 L340 L341 L342 L343 L344 L345 L346 L347 L348 L349 L350 L351 L352 L353 L354 L355 L356 L357 L358 L359 L360 L361 L362 L363 L364 L365 L366 L367 L368 L369 L370 L371 L372 L373 L374 L375 L376 L377 L378 L379 L380 L381 L382 L383 L384 L385 L386 L387 L388 L389 L390 L391 L392 L393 L394 L395 L396 L397 L398 L399 L400 L401 L402 L403 L404 L405 L406 L407 L408 L409 L410 L411 L412 L413 L414 L415 L416 L417 L418 L419 L420 L421 L422 L423 L424 L425 L426 L427 L428 L429 L430 L431 L432 L433 L434 L435 L436 L437 L438 L439 L440 L441 L442 L443 L444 L445 L446 L447 L448 L449 L450 L451 L452 L453 L454 L455 L456 L457 L458 L459 L460 L461 L462 L463 L464 L465 L466 L467 L468 L469 L470 L471 L472 L473 L474 L475 L476 L477 L478 L479 L480 L481 L482 L483 L484 L485 L486 L487 L488 L489 L490 L491 L492 L493 L494 L495 L496 L497 L498 L499 L500 L501 L502 L503 L504 L505 L506 L507 L508 L509 L510 L511 L512 L513 L514 L515 L516 L517 L518 L519 L520 L521 L522 L523 L524 L525 L526 L527 L528 L529 L530 L531 L532 L533 L534 L535 L536 L537 L538 L539 L540 L541 L542 L543 L544 L545 L546 L547 L548 L549 L550 L551 L552 L553 L554 L555 L556 L557 L558 L559 L560 L561 L562 L563 L564 L565 L566 L567 L568 L569 L570 L571 L572 L573 L574 L575 | L576 L577 A0 | A0 L577 L576 | L577 L576 A0 | A0 L576 L577
sketch "Эскиз2" plane through (0, 0, 5) normal (0, 0, 1) x (1, 0, 0)
  line L0 (0.0073, 17.4785) -> (0.0073, 16.4837) projected
  line L1 (0.0073, 16.9811) -> (33.9549, 16.9811)
  line L2 (33.9549, 16.4837) -> (33.9549, 17.4785) projected
  circle A0 centre (16.9811, 16.9811) radius 12.5
  point P0 (0, 0)
  dimension "d2" = 25
  constraints: 3 midpoint, 2 end point, 1 centre point
  measures "d2" diameter of A0
extrude "Выдавливание2" add sketch "Эскиз2" along normal blind 13
sketch "Эскиз4" plane through (0, 0, 0) normal (0, 0, -1) x (-1, 0, 0)
  circle A0 centre (-16.9811, 16.9811) radius 12.5 projected
  circle A1 centre (-16.9811, 16.9811) radius 5
  point P0 (0, 0)
  dimension "d5" = 10
  constraints: 1 centre point, 1 coincident
  measures "d5" diameter of A1
extrude "Выдавливание3" add sketch "Эскиз4" along normal blind 16 contours A1
sketch "Эскиз5" plane through (16.9811, 16.9811, -16) normal (0, 0, -1) x (-1, 0, 0)
  circle A0 centre (0, 0) radius 5 projected
  point P0 (16.9811, -16.9811)
hole "Отверстие1" at (16.9811, 16.9811, -16) direction (0, 0, 1) diameter 9 depth 8 tip angle 118
sketch "Эскиз6" plane through (16.9811, 16.9811, -16) normal (0, 0, -1) x (-1, 0, 0)
  line L0 (-5, 1) -> (5, 1)
  line L1 (5, 1) -> (5, -1)
  line L2 (5, -1) -> (-5, -1)
  line L3 (-5, -1) -> (-5, 1)
  line L4 (-5, 1) -> (5, -1) construction
  line L5 (5, 1) -> (-5, -1) construction
  circle A0 centre (0, 0) radius 5 projected
  point P0 (16.9811, -16.9811)
  point P1 (0, 0)
  dimension "d15" = 2
  constraints: 12 end point, 3 midpoint, 2 parallel, 2 tangent, 1 coincident, 1 horizontal, 1 perpendicular
  measures "d15" distance of L0.end L1.end
extrude "Выдавливание4" cut sketch "Эскиз6" against normal up to surface contours L0 A0 L3 | L0 A0 L2 | A0 L2 L3 | L0 L1 A0 | L1 L2 A0 round surface about axis through (16.9811, 16.9811, -6.6481) along (0, 0, -1) radius 2.25 half angle 59 far side no
ref_plane "РабПлоскость1" through (16.9811, 16.9811, 9) normal (0, 0, 1) x (1, 0, 0)
mirror "Зеркальное отражение1" about plane through (16.9811, 16.9811, 9) normal (0, 0, 1) of "Выдавливание3", "Отверстие1", "Выдавливание4"
fillet "Сопряжение1" radius 1 1 edges at (4.4811, 16.9811, 18)
